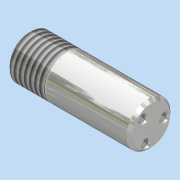
# Autodesk Inventor part: Überlast Führung
Saved by Autodesk Inventor 2021 (Build 250183000, 183)
## iProperties
Created: 2024-03-14
Part Number: Überlast Führung
Material: Generic
Document SubType Name: Modeling
Designer: Nokia
Density: 1 g/cm^3
Appearance: Aluminum - Dark
Author: Nokia
Autodesk Inventor part; units mm, degrees
ref_plane "YZ Plane" through (0, 0, 0) normal (1, 0, 0) x (0, 1, 0)
ref_plane "XZ Plane" through (0, 0, 0) normal (0, 1, 0) x (-1, 0, 0)
ref_plane "XY Plane" through (0, 0, 0) normal (0, 0, 1) x (1, 0, 0)
sketch "Sketch1" plane through (0, 0, 0) normal (0, 0, 1) x (1, 0, 0)
  line L0 (0, 0) -> (0, 15)
  line L1 (-84, 15) -> (-84, 0)
  line L2 (-84, 0) -> (0, 0)
  arc A0 (-58, 15) -> (-57, 15) centre (-57.5, 15) ccw
  line L3 (0, 15) -> (-57, 15)
  line L4 (-58, 15) -> (-84, 15)
  dimension "d0" = 15
  dimension "d1" = 84
  constraints: 10 end point, 5 perpendicular, 2 point on circle, 1 centre point, 1 vertical
  measures "d0" distance of L0.start L0.end
  measures "d1" distance of L0.end L1.start
revolve "Revolution1" add sketch "Sketch1" angle 360 about axis through (-84, 0, 0) along (1, 0, 0)
thread "Thread1" size "M30x3.5" class "6g" standard "ANSI Metric M Profile" length 50
sketch "Sketch2" plane through (0, 0, 0) normal (1, 0, 0) x (0, 0, -1)
  circle A0 centre (0, 0) radius 15
  circle A1 centre (9, 0) radius 3.5
  circle A2 centre (-4.5, 7.7942) radius 3.5
  circle A3 centre (-4.5, -7.7942) radius 3.5
  dimension "d10" = 30
  dimension "d11" = 7
  dimension "d12" = 360
  dimension "d13" = 9
  dimension "d27" = 0
  dimension "d28" = 0
  dimension "d29" = 0
  constraints: 4 centre point, 1 coincident, 7 other
  measures "d10" diameter of A0
  measures "d11" diameter of A1
  measures "d13" distance of A1.centre point (0, 0)
  measures "d27" distance of point (0, 0) point (0, 0)
  measures "d28" distance of point (0, 0) point (0, 0)
  measures "d29" vertical distance of point (0, 0) A1.centre
hole "Hole1" at (0, 0, -9) at (0, 7.7942, 4.5) at (0, -7.7942, 4.5) direction (-1, 0, 0) diameter 4.917 depth 28 tip angle 118 thread size "M6x1" class "6H" standard "ISO Metric profile"
chamfer "Chamfer1" distance 2 angle 45 2 edges at (-84, -15, 0) (0, -15, 0)
chamfer "Chamfer2" distance 1 angle 45 3 edges at (0, 0, -6.5415) (0, -7.7942, 6.9585) (0, 7.7942, 6.9585)
body "Solid1"
